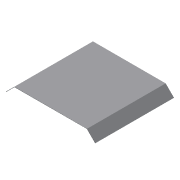
# Autodesk Inventor part: LoadSlide
Saved by Autodesk Inventor 2015 (Build 190159000, 159)
## iProperties
Created: 2015-03-06
Part Number: LoadSlide
Material: Polycarbonate, Clear
Document SubType Name: Modeling
Designer: Jaden
Density: 1.2 g/cm^3
Appearance: Polycarbonate - Clear
Author: Jaden
Autodesk Inventor part; units mm, degrees
ref_plane "YZ Plane" through (0, 0, 0) normal (1, 0, 0) x (0, 1, 0)
ref_plane "XZ Plane" through (0, 0, 0) normal (0, 1, 0) x (-1, 0, 0)
ref_plane "XY Plane" through (0, 0, 0) normal (0, 0, 1) x (1, 0, 0)
sketch "Sketch1" plane through (0, 0, 0) normal (0, 0, 1) x (1, 0, 0)
  line L0 (0, 0) -> (53.8815, 53.8815)
  line L1 (0, 0) -> (76.2, 0) construction
  line L2 (0, 0) -> (1.4368, -1.4368)
  line L3 (53.8815, 53.8815) -> (523.7815, 53.8815) construction
  line L4 (523.7815, 53.8815) -> (577.6409, -0.0222)
  line L5 (577.6409, -0.0222) -> (576.2034, -1.4585)
  line L6 (523.7815, 53.8815) -> (525.8135, 53.8815) construction
  line L7 (522.3441, 52.4453) -> (576.2034, -1.4585)
  line L8 (53.8815, 51.8495) -> (1.4368, -1.4368)
  line L9 (53.8815, 51.8495) -> (522.3441, 52.4453)
  line L10 (53.8815, 53.8815) -> (523.7815, 53.8815)
  dimension "d0" = 76.2
  dimension "d1" = 45
  dimension "d2" = 2.032
  dimension "d5" = 76.2
  dimension "d6" = 2.032
  dimension "d7" = 2.032
  dimension "d9" = 2.032
  constraints: 22 end point, 4 horizontal, 1 equal length, 1 parallel, 1 perpendicular
  measures "d0" distance of L0.start L0.end
  measures "d1" angle of L1 L0
  measures "d2" distance of L0.start L2.end
  measures "d5" distance of L3.end L4.end
  measures "d6" distance of L4.end L5.end
  measures "d7" distance of L3.end L7.start
  measures "d9" distance of L0.end L8.start
extrude "Extrusion1" add sketch "Sketch1" along normal blind 508
body "Solid1"
